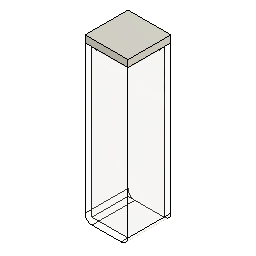
Quartz Couvette v1 (Autodesk Fusion 360 design; units mm, degrees)
Autodesk Fusion 360 part; units mm, degrees
sketch "Sketch1" plane through (0, 0, 0) normal (0, 0, 1) x (1, 0, 0)
sketch "Sketch2" plane through (0, 0, 0) normal (0, 0, 1) x (1, 0, 0)
box "BoxPrimitive1" add length 12.5 width 12.5 height 45 placed x (0, 1, 0) y (-1, 0, 0) z (0, 0, 1) at (12.5, 0, 0) makes body 1
shell "Shell1" thickness 1 removed faces 1 at (4.1667, 4.1667, 45) on bodies 1
fillet "Fillet1" radius 2 2 edges at (0, 6.25, 0) (12.5, 6.25, 0) on bodies 1
box "BoxPrimitive2" add length 12.5 width 12.5 height 2 placed x (0, 1, 0) y (-1, 0, 0) z (0, 0, 1) at (5.6776, 0, 0) separate body makes body 2
box "BoxPrimitive3" add length 9.5 width 9.5 height 2 placed x (0, -1, 0) y (1, 0, 0) z (0, 0, 1) at (-4, 9, 2) separate body makes body 3
move_body "Align1" bodies 3 to x (1, 0, 0) y (0, -1, 0) z (0, 0, -1) at (-1.3224, 10.5, 6)
box "BoxPrimitive4" add length 7.5 width 7.5 height 2 placed x (0, -1, 0) y (1, 0, 0) z (0, 0, 1) at (-4, 9.5, 4) separate body makes body 4
move_body "Align2" bodies 4 to x (1, 0, 0) y (0, 1, 0) z (0, 0, 1) at (-0.3224, 0.5, -2)
combine "Combine1" operation cut target body 3 tool bodies 4
fillet "Fillet2" radius 0.5 4 edges at (4.1776, 6.25, 4) (-0.5724, 1.5, 4) (-5.3224, 6.25, 4) (-0.5724, 11, 4) on bodies 3
combine "Combine2" operation add target body 2 tool bodies 3
move_body "Move1" bodies 2 to x (1, 0, 0) y (0, -1, 0) z (0, 0, -1) at (0, 0, 0)
move_body "Move2" bodies 2 to x (1, 0, 0) y (0, 1, 0) z (0, 0, 1) at (1, 6, 0)
move_body "Move3" bodies 2 to x (1, 0, 0) y (0, 1, 0) z (0, 0, 1) at (-0.4276, 0.25, 0)
copy_body "Body->Comp1" bodies 2 removing the originals makes body 5 in component "Couvette Lid"
move_body "Move4" bodies 1 to x (1, 0, 0) y (0, 1, 0) z (0, 0, 1) at (-6.25, -6.25, 0)
copy_body "Body->Comp2" bodies 1 removing the originals makes body 6 in component "Couvette 12.5x12.5x45"
move_body "Align1'" bodies 5 to x (1, 0, 0) y (0, 1, 0) z (0, 0, 1) at (0, 0, 47) in component "Couvette Lid"
component "Couvette Lid" placed x (1, 0, 0) y (0, 1, 0) z (0, 0, 1) at (0, 0, 0)
component "Couvette 12.5x12.5x45" placed x (1, 0, 0) y (0, 1, 0) z (0, 0, 1) at (0, 0, 0)
